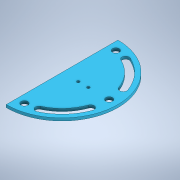
# Autodesk Inventor part: Base 3
Saved by Autodesk Inventor 2020 (Build 240168000, 168)
## iProperties
Created: 2020-10-28
Part Number: Base 3
Material: PC/ABS Plastic
Document SubType Name: Modeling
Designer: aaron
Density: 0.357273 g/cm^3
Appearance: Turquoise
Author: aaron
## iProperties of the stored document _3DPrint.ipt
Created: 2020-11-03
Part Number: _3DPrint
Material: Generic
Document SubType Name: Modeling
Designer: aaron
Density: 1 g/cm^3
Appearance: Default
Author: aaron
Autodesk Inventor part; units mm, degrees
ref_plane "YZ Plane" through (0, 0, 0) normal (1, 0, 0) x (0, 1, 0)
ref_plane "XZ Plane" through (0, 0, 0) normal (0, 1, 0) x (-1, 0, 0)
ref_plane "XY Plane" through (0, 0, 0) normal (0, 0, 1) x (1, 0, 0)
sketch "Sketch1" plane through (0, 0, 0) normal (0, 1, 0) x (-1, 0, 0)
  circle A0 centre (0, 0) radius 41.5 construction
  line L0 (0, -41.5) -> (0, 41.5)
  arc A1 (0, 41.5) -> (0, -41.5) centre (0, 0) ccw
  circle A2 centre (-6, -34) radius 2.5
  circle A3 centre (-6, 34) radius 2.5
  line L1 (0, 0) -> (-41.5, 0) construction
  circle A4 centre (-35, 0) radius 2.5
  circle A5 centre (0, 0) radius 35.5 construction
  line L2 (0, 0) -> (-38.9972, -14.1938) construction
  line L3 (0, 0) -> (-17.5387, -37.6118) construction
  arc A6 (-33.3591, -12.1417) -> (-15.0029, -32.1739) centre (0, 0) ccw construction
  arc A7 (-35.8493, -13.0481) -> (-16.1229, -34.5756) centre (0, 0) ccw
  arc A8 (-30.8689, -11.2354) -> (-13.883, -29.7722) centre (0, 0) ccw
  arc A9 (-30.8689, -11.2354) -> (-35.8493, -13.0481) centre (-33.3591, -12.1417) ccw
  arc A10 (-16.1229, -34.5756) -> (-13.883, -29.7722) centre (-15.0029, -32.1739) ccw
  arc A11 (-16.1229, 34.5756) -> (-35.8493, 13.0481) centre (0, 0) ccw
  arc A12 (-13.883, 29.7722) -> (-30.8689, 11.2354) centre (0, 0) ccw
  arc A13 (-35.8493, 13.0481) -> (-30.8689, 11.2354) centre (-33.3591, 12.1417) ccw
  arc A14 (-13.883, 29.7722) -> (-16.1229, 34.5756) centre (-15.0029, 32.1739) ccw
  dimension "d0" = 83
  dimension "d1" = 83
  dimension "d2" = 5
  dimension "d3" = 6
  dimension "d4" = 34
  dimension "d5" = 34
  dimension "d6" = 35
  dimension "d7" = 6
  dimension "d8" = 20
  dimension "d9" = 25
  dimension "d10" = 5.3
  constraints: 27 point on circle, 15 centre point, 8 end point, 6 symmetric about line, 4 equal radius, 4 tangent, 3 point on line, 2 coincident, 1 concentric, 1 midpoint, 1 vertical, 1 vertical alignment, 4 other
  measures "d0" diameter of A0
  measures "d1" distance of L0.start L0.end
  measures "d2" diameter of A2
  measures "d3" horizontal distance of point (0, 0) A2.centre
  measures "d4" vertical distance of point (0, 0) A2.centre
  measures "d5" vertical distance of point (0, 0) A3.centre
  measures "d6" distance of point (0, 0) A4.centre
  measures "d7" radial gap between concentric circles of A0 A5
  measures "d8" angle of L2 L1
  measures "d9" angle of L0 L3
  measures "d10" diameter of A10
extrude "Extrusion1" add sketch "Sketch1" along normal blind 2
sketch "Sketch2" plane through (0, 2, 0) normal (0, 1, 0) x (1, 0, 0)
  arc A0 (0, -41.5) -> (0, 41.5) centre (0, 0) ccw construction
  circle A1 centre (12, 0) radius 1
  circle A2 centre (19.5, 0) radius 1
  line L0 (0, 0) -> (41.5, 0) construction
  dimension "d13" = 7.5
  dimension "d14" = 2
  dimension "d15" = 12
  constraints: 2 centre point, 2 end point, 2 point on line, 1 equal radius, 1 point on circle
  measures "d13" distance of A2.centre A1.centre
  measures "d14" diameter of A2
  measures "d15" distance of point (0, 0) A1.centre
extrude "Extrusion2" cut sketch "Sketch2" against normal through all
body "Solid1"
